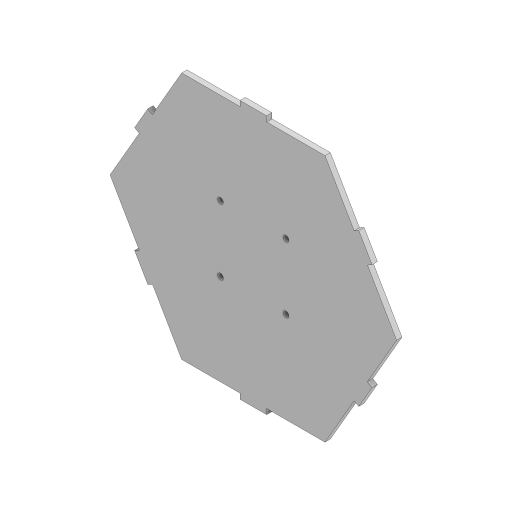
# Autodesk Inventor part: middle_space2
Saved by Autodesk Inventor 2024 (Build 280153000, 153)
## iProperties
Created: 2024-03-28
Part Number: middle_space2
Material: Generic
Document SubType Name: Modeling
Designer: op04o
Density: 1 g/cm^3
Appearance: Default
Author: op04o
Autodesk Inventor part; units mm, degrees
ref_plane "YZ Plane" through (0, 0, 0) normal (1, 0, 0) x (0, 1, 0)
ref_plane "XZ Plane" through (0, 0, 0) normal (0, 1, 0) x (-1, 0, 0)
ref_plane "XY Plane" through (0, 0, 0) normal (0, 0, 1) x (1, 0, 0)
sketch "Sketch1" plane through (0, 0, 0) normal (0, 0, 1) x (1, 0, 0)
  line L0 (-7.5, 73) -> (7.5, 73)
  line L1 (7.5, 73) -> (7.5, 70)
  line L2 (-7.5, 70) -> (-7.5, 73)
  line L3 (-40.4145, 70) -> (-7.5, 70)
  line L4 (7.5, 70) -> (40.4145, 70)
  line L5 (-66.9699, 30.0048) -> (-59.4699, 42.9952)
  line L6 (-59.4699, 42.9952) -> (-56.8718, 41.4952)
  line L7 (-64.3718, 28.5048) -> (-66.9699, 30.0048)
  line L8 (-59.4699, -42.9952) -> (-66.9699, -30.0048)
  line L9 (-66.9699, -30.0048) -> (-64.3718, -28.5048)
  line L10 (-56.8718, -41.4952) -> (-59.4699, -42.9952)
  line L11 (7.5, -73) -> (-7.5, -73)
  line L12 (-7.5, -73) -> (-7.5, -70)
  line L13 (7.5, -70) -> (7.5, -73)
  line L14 (66.9699, -30.0048) -> (59.4699, -42.9952)
  line L15 (59.4699, -42.9952) -> (56.8718, -41.4952)
  line L16 (64.3718, -28.5048) -> (66.9699, -30.0048)
  line L17 (59.4699, 42.9952) -> (66.9699, 30.0048)
  line L18 (66.9699, 30.0048) -> (64.3718, 28.5048)
  line L19 (56.8718, 41.4952) -> (59.4699, 42.9952)
  line L20 (-80.829, 0) -> (-64.3718, 28.5048)
  line L21 (-56.8718, 41.4952) -> (-40.4145, 70)
  line L22 (40.4145, 70) -> (56.8718, 41.4952)
  line L23 (64.3718, 28.5048) -> (80.829, 0)
  line L24 (80.829, 0) -> (64.3718, -28.5048)
  line L25 (56.8718, -41.4952) -> (40.4145, -70)
  line L26 (40.4145, -70) -> (7.5, -70)
  line L27 (-7.5, -70) -> (-40.4145, -70)
  line L28 (-40.4145, -70) -> (-56.8718, -41.4952)
  line L29 (-64.3718, -28.5048) -> (-80.829, 0)
  circle A0 centre (-18.5, 18.5) radius 1.6
  circle A1 centre (18.5, 18.5) radius 1.6
  circle A2 centre (18.5, -18.5) radius 1.6
  circle A3 centre (-18.5, -18.5) radius 1.6
  point P0 (0, 0)
  point P1 (0, 0)
  point P2 (0, 73)
  point P3 (-63.2199, 36.5)
  point P4 (-63.2199, -36.5)
  point P5 (0, -73)
  point P6 (63.2199, -36.5)
  point P7 (63.2199, 36.5)
  dimension "d1" = 3
  dimension "d3" = 15
  dimension "d6" = 360
  dimension "d8" = 140
  dimension "d9" = 146
  dimension "d12" = 3.2
  dimension "d13" = 3.2
  dimension "d14" = 3.2
  dimension "d15" = 3.2
  dimension "d16" = 37
  dimension "d17" = 37
  dimension "d18" = 18.5
  dimension "d19" = 18.5
  constraints: 60 end point, 4 centre point, 3 horizontal, 3 vertical alignment, 2 horizontal alignment, 1 coincident, 1 midpoint, 1 parallel, 1 perpendicular, 56 other
  measures "d1" distance of L2.start L0.start
  measures "d3" distance of L0.start L0.end
  measures "d8" distance between parallel lines of L27 L3
  measures "d9" distance between parallel lines of L14 L5
  measures "d12" diameter of A0
  measures "d13" diameter of A1
  measures "d14" diameter of A2
  measures "d15" diameter of A3
  measures "d16" distance of A2.centre A3.centre
  measures "d17" distance of A2.centre A1.centre
  measures "d18" horizontal distance of point (0, 0) A3.centre
  measures "d19" horizontal distance of point (0, 0) A1.centre
extrude "Extrusion2" add sketch "Sketch1" along normal blind 3
body "Solid2"
